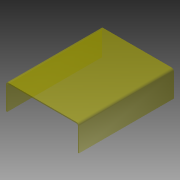
# Autodesk Inventor part: shield2a
Saved by Autodesk Inventor 2014 SP2 (Build 180246200, 246)
## iProperties
Created: 2016-10-05
Part Number: shield2a
Material: Generic
Document SubType Name: Sheet Metal
Designer: cruiser
Density: 1 g/cm^3
Sheet Metal Rule: Default_mm
Appearance: Clear - Yellow
Flat Pattern Width: 26.0794 cm
Flat Pattern Length: 33.1486 cm
Flat Pattern Area: 864.496 cm^2
Sheet Metal Width: 260.794 mm
Sheet Metal Length: 331.486 mm
Sheet Metal Area: 86449.603 mm^2
Author: cruiser
Autodesk Inventor part; units mm, degrees
ref_plane "YZ Plane" through (0, 0, 0) normal (1, 0, 0) x (0, 1, 0)
ref_plane "XZ Plane" through (0, 0, 0) normal (0, 1, 0) x (-1, 0, 0)
ref_plane "XY Plane" through (0, 0, 0) normal (0, 0, 1) x (1, 0, 0)
sketch "Sketch1" plane through (0, 0, 0) normal (0, 0, 1) x (1, 0, 0)
  line L0 (-100.2181, -130.3969) -> (100.2181, -130.3969)
  line L1 (100.2181, -130.3969) -> (100.2181, 130.3969)
  line L2 (100.2181, 130.3969) -> (-100.2181, 130.3969)
  line L3 (-100.2181, 130.3969) -> (-100.2181, -130.3969)
  line L4 (-100.2181, -130.3969) -> (100.2181, 130.3969) construction
  line L5 (100.2181, -130.3969) -> (-100.2181, 130.3969) construction
  point P0 (0, 0)
  dimension "d0" = 200.4362
  dimension "d1" = 260.7937
  measures "d0" distance of L2.end L1.end
  measures "d1" distance of L1.end L0.end
extrude "Plate1" add sketch "Sketch1" along normal blind 3.15
sketch "Sketch2" plane through (97.0681, -130.3969, 3.15) normal (1, 0, 0) x (0, 1, 0)
  line L0 (260.7937, 0) -> (0, 0)
  line L1 (0, 0) -> (0, -71)
  line L2 (0, -71) -> (260.7937, -71)
  line L3 (260.7937, -71) -> (260.7937, 0)
  constraints: 6 end point, 1 horizontal, 1 perpendicular, 1 vertical
edge flange "Flange1" height 71 angle 90 thickness 3.15 bend radius 3.15 thickness toward (1, 0, 0) relief straight relief width 3.15 relief depth 1.575 corner gap 3.15 corner form 0 edges at (100.2181, 0, 0) (-100.2181, 0, 0) wall of the first edge with corners at (97.0681, 130.3969, 3.15) (97.0681, -130.3969, 3.15) (97.0681, -130.3969, -67.85) (97.0681, 130.3969, -67.85)
bend "Bend1"
corner "Corner1"
equation "\"d0\" = shield_x"
equation "\"d1\" = shield_z"
equation "\"Thickness\" = shield_t"
equation "\"d3\" = BendReliefWidth"
equation "\"d4\" = BendReliefDepth"
equation "\"d5\" = MinimumRemnant"
equation "\"d6\" = BendRadius"
equation "\"d7\" = shield_y"
equation "\"d9\" = BendRadius"
equation "\"d10\" = CornerReliefSize"
equation "\"d11\" = GapSize"
equation "\"d12\" = JacobiRadiusSize"
equation "\"BendRadius\" = Thickness"
equation "\"BendReliefWidth\" = Thickness"
equation "\"BendReliefDepth\" = 0.5 * Thickness"
equation "\"CornerReliefSize\" = 4 * Thickness"
equation "\"MinimumRemnant\" = 2 * Thickness"
equation "\"TransitionRadius\" = BendRadius"
equation "\"JacobiRadiusSize\" = BendRadius"
equation "\"GapSize\" = Thickness"
equation "\"laserresin\" = 5"
equation "\"st1_thickness\" = 0.91186"
equation "\"st2_thickness\" = 1.5875"
equation "\"st3_thickness\" = 1.5875"
equation "\"al1_thickness\" = 0.79375"
equation "\"al2_thickness\" = 1.5875"
equation "\"al3_thickness\" = 1.5875"
equation "\"bend_factor\" = 2.26205"
equation "\"st1_bend\" = 2.06267"
equation "\"st2_bend\" = 3.591"
equation "\"st3_bend\" = 3.591"
equation "\"al1_bend\" = 1.7955"
equation "\"al2_bend\" = 3.591"
equation "\"al3_bend\" = 3.591"
equation "\"acrylic1_thickness\" = 5.88"
equation "\"acrylic2_thickness\" = 3.15"
equation "\"acrylic3_thickness\" = 3.15"
equation "\"corner_small_r\" = 1"
equation "\"corner_big_r\" = 5"
equation "\"linear_bearing_spacing\" = 209"
equation "\"galvo_y_out_offset\" = 27"
equation "\"galvo_y_in_offset\" = 17.5"
equation "\"laser_diameter\" = 13"
equation "\"nema17_x\" = 43"
equation "\"nema17_shaft\" = 24"
equation "\"lmk8uu_x\" = 25"
equation "\"lmk8uu_shaft\" = 15"
equation "\"lmk8uu_z\" = 24"
equation "\"shf8_y\" = 43"
equation "\"acme_nut_d\" = 19.1"
equation "\"acme_nut_upper_d\" = 12.7"
equation "\"handle_spacing\" = 50.8"
equation "\"handle_d\" = 4.7625"
equation "\"handle_hole_d\" = 5.0625"
equation "\"handle_projection\" = 20.6375"
equation "\"switch_spacing\" = 19"
equation "\"laser_body_diameter\" = 12"
equation "\"m3_diameter\" = 3"
equation "\"m3_head\" = 6"
equation "\"m4_diameter\" = 4"
equation "\"m5_diameter\" = 5"
equation "\"m5_head\" = 10.3"
equation "\"rivet1_diameter\" = 3.26"
equation "\"rivet2_diameter\" = 3.26"
equation "\"brass_insert_drill\" = 4"
equation "\"m5_brass_insert_drill\" = 6.7"
equation "\"m3_press_nut_drill\" = 4.5"
equation "\"m5_press_nut_drill\" = 6.5"
equation "\"platform_t\" = 1.5875"
equation "\"platform_z\" = 65"
equation "\"platform_fold_x\" = 15"
equation "\"platform_crane_gap\" = 0.1"
equation "\"platform_gap\" = 0.1"
equation "\"platform_upper_y\" = 46.625"
equation "\"crane_t\" = 1.5875"
equation "\"crane_x\" = 234"
equation "\"crane_gap\" = 0.1"
equation "\"tray_t\" = 5.88"
equation "\"tray_to_platform_oversize\" = 0"
equation "\"reservoir_t\" = 0.79375"
equation "\"reservoir_z\" = 35"
equation "\"reservoir_flap_y\" = 20.79375"
equation "\"frame_front_t\" = 0.91186"
equation "\"frame_front_x\" = 280.23622"
equation "\"frame_front_y\" = 56"
equation "\"frame_front_fold\" = 15"
equation "\"frame_gap\" = 0.1"
equation "\"frame_back_t\" = 0.91186"
equation "\"frame_back_x\" = 278.2125"
equation "\"frame_back_y\" = 53.97628"
equation "\"frame_back_z\" = 497.97628"
equation "\"frame_opening_x\" = 200.23622"
equation "\"drawer_t\" = 0.79375"
equation "\"drawer_gap\" = 0.1"
equation "\"drawer_reservoir_overlap_x\" = 24.20625"
equation "\"drawer_x\" = 202.02372"
equation "\"drawer_y\" = 73"
equation "\"drawer_seal_y\" = 101"
equation "\"drawer_window_gap\" = 6"
equation "\"foot_t\" = 1.5875"
equation "\"foot_x\" = 199"
equation "\"foot_y\" = 196"
equation "\"laser_holder_t\" = 0.79375"
equation "\"laser_holder_z\" = 75"
equation "\"laser_offset_x\" = 59.5"
equation "\"laser_offset_y\" = 8.5"
equation "\"subframe_t\" = 0.79375"
equation "\"subframe_x\" = 66"
equation "\"subframe_y\" = 55"
equation "\"shield_t\" = 3.15"
equation "\"shield_x\" = 200.43622"
equation "\"shield_y\" = 71"
equation "\"shield_z\" = 260.79375"
equation "\"magnet_t\" = 1.6"
equation "\"magnet_w\" = 12.8"
equation "\"d2\" = BendRadius"
body "Solid1"
